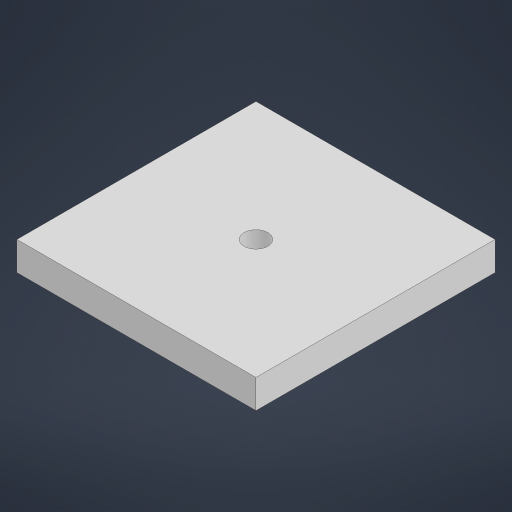
# Autodesk Inventor part: Manual_NC_REF
Saved by Autodesk Inventor 2024.3 (Build 283343000, 343)
## iProperties
Created: 2023-09-10
Part Number: Manual_NC_REF
Material: Generic
Document SubType Name: Modeling
Designer: Benjamin
Density: 1 g/cm^3
Appearance: Default
Author: Benjamin
Autodesk Inventor part; units mm, degrees
ref_plane "YZ Plane" through (0, 0, 0) normal (1, 0, 0) x (0, 1, 0)
ref_plane "XZ Plane" through (0, 0, 0) normal (0, 1, 0) x (-1, 0, 0)
ref_plane "XY Plane" through (0, 0, 0) normal (0, 0, 1) x (1, 0, 0)
sketch "Sketch1" plane through (0, 0, 0) normal (0, 1, 0) x (-1, 0, 0)
  line L0 (70, 0) -> (-70, 0) construction
  line L1 (0, -70) -> (0, 70) construction
  line L2 (-50, 50) -> (50, 50)
  line L3 (50, 50) -> (50, -50)
  line L4 (50, -50) -> (-50, -50)
  line L5 (-50, -50) -> (-50, 50)
  line L6 (-50, 50) -> (50, -50) construction
  line L7 (50, 50) -> (-50, -50) construction
  circle A0 centre (0, 0) radius 5
  dimension "d0" = 100
  dimension "d3" = 10
  constraints: 12 end point, 2 midpoint, 2 parallel, 2 perpendicular, 1 centre point, 1 coincident, 1 horizontal
  measures "d0" distance of L3.end L4.end
  measures "d3" diameter of A0
extrude "Extrusion1" add sketch "Sketch1" along normal blind 12
body "Solid1"
